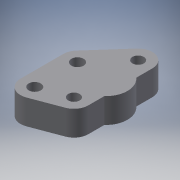
# Autodesk Inventor part: BLTouch_Connector
Saved by Autodesk Inventor 2016 (Build 200138000, 138)
## iProperties
Created: 2015-12-28
Part Number: BLTouch_Connector
Material: Generic
Document SubType Name: Modeling
Designer: inornate
Density: 1 g/cm^3
Appearance: Default
Author: inornate
Autodesk Inventor part; units mm, degrees
ref_plane "YZ Plane" through (0, 0, 0) normal (1, 0, 0) x (0, 1, 0)
ref_plane "XZ Plane" through (0, 0, 0) normal (0, 1, 0) x (-1, 0, 0)
ref_plane "XY Plane" through (0, 0, 0) normal (0, 0, 1) x (1, 0, 0)
sketch "Sketch1" plane through (0, 0, 0) normal (0, 0, 1) x (1, 0, 0)
  circle A0 centre (22, -5.4955) radius 1.7 projected
  circle A1 centre (22, 6.5045) radius 1.7 projected
  arc A2 (22, -9.4955) -> (26, -5.4955) centre (22, -5.4955) ccw construction
  line L0 (22, -5.4955) -> (22, 6.5045) construction
  line L1 (18, 6.5045) -> (18, -5.4955)
  arc A3 (18, -5.4955) -> (23.4045, -9.2408) centre (22, -5.4955) ccw
  circle A4 centre (30, 15.5045) radius 1.6
  circle A5 centre (30, -2.4955) radius 1.6
  arc A6 (34, 15.5045) -> (27.0104, 18.162) centre (30, 15.5045) ccw
  arc A7 (31.4045, -6.2408) -> (34, -2.4955) centre (30, -2.4955) ccw
  line L2 (34, -2.4955) -> (34, 2.0324)
  line L3 (34, 10.9767) -> (34, 15.5045)
  arc A8 (34, 2.0324) -> (34, 10.9767) centre (30, 6.5045) ccw
  line L4 (19.0104, 9.162) -> (27.0104, 18.162)
  arc A9 (19.0104, 9.162) -> (18, 6.5045) centre (22, 6.5045) ccw
  line L5 (23.4045, -9.2408) -> (31.4045, -6.2408)
  circle A10 centre (22, -5.4955) radius 1.7 projected
  circle A11 centre (-15, -5.4955) radius 1.7 projected
  circle A12 centre (-15, 6.5045) radius 1.7 projected
  circle A13 centre (22, 6.5045) radius 1.7 projected
  circle A14 centre (-8, 6.5045) radius 1.7 projected
  arc A15 (-15, 10.5045) -> (-19, 6.5045) centre (-15, 6.5045) ccw projected
  line L6 (-19, 6.5045) -> (-19, -5.4955) projected
  arc A16 (-19, -5.4955) -> (-15, -9.4955) centre (-15, -5.4955) ccw projected
  line L7 (-15, -9.4955) -> (22, -9.4955) projected
  arc A17 (22, -9.4955) -> (26, -5.4955) centre (22, -5.4955) ccw projected
  line L8 (26, -5.4955) -> (26, 6.5045) projected
  arc A18 (26, 6.5045) -> (22, 10.5045) centre (22, 6.5045) ccw projected
  line L9 (22, 10.5045) -> (15.2, 10.5045) projected
  arc A19 (15.2, 10.5045) -> (13.2, 8.5045) centre (15.2, 8.5045) ccw projected
  line L10 (13.2, 8.5045) -> (13.2, 6.5045) projected
  arc A20 (0.8, 6.5045) -> (13.2, 6.5045) centre (7, 6.5045) ccw projected
  line L11 (0.8, 6.5045) -> (0.8, 8.5045) projected
  arc A21 (0.8, 8.5045) -> (-1.2, 10.5045) centre (-1.2, 8.5045) ccw projected
  line L12 (-1.2, 10.5045) -> (-15, 10.5045) projected
  line L13 (30, 15.5045) -> (30, -2.4955) construction
  circle A22 centre (30, 6.5045) radius 2.5
  point P0 (22, 0.5045)
  dimension "d5" = 8
  dimension "d7" = 8
  dimension "d8" = 6
  dimension "d10" = 3.2
  dimension "d11" = 4
  dimension "d15" = 18
  dimension "d16" = 5
  constraints: 16 end point, 11 point on circle, 10 tangent, 8 centre point, 2 coincident, 2 midpoint, 1 concentric, 1 horizontal alignment, 1 perpendicular
  measures "d5" diameter of A7
  measures "d7" horizontal distance of L13.end A0.centre
  measures "d8" radius of A8
  measures "d10" diameter of A4
  measures "d11" radius of A6
  measures "d15" distance of L13.start L13.end
  measures "d16" diameter of A22
extrude "Extrusion1" add sketch "Sketch1" along normal blind 7 contours A9 L4 L9 A18 L8 A17 A3 L1 | L4 A6 L3 A8 L2 A7 L5 A17 L8 A18 L9 | A22
body "Solid1"
